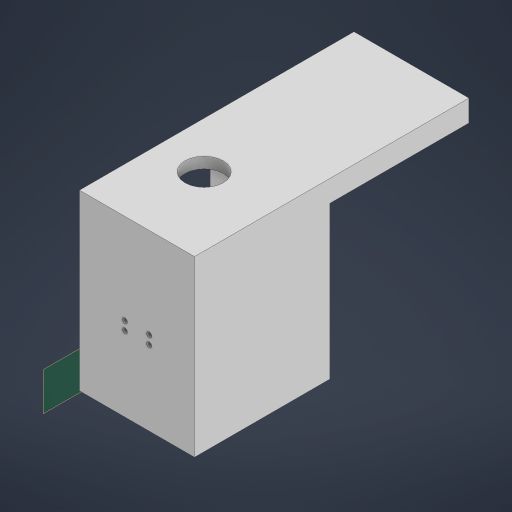
# Autodesk Inventor part: Gearbox
Saved by Autodesk Inventor 2024 (Build 280153000, 153)
## iProperties
Created: 2024-03-09
Part Number: Gearbox
Material: Generic
Document SubType Name: Modeling
Designer: LightStore
Density: 1 g/cm^3
Appearance: Default
Author: LightStore
Autodesk Inventor part; units mm, degrees
ref_plane "YZ Plane" through (0, 0, 0) normal (1, 0, 0) x (0, 1, 0)
ref_plane "XZ Plane" through (0, 0, 0) normal (0, 1, 0) x (-1, 0, 0)
ref_plane "XY Plane" through (0, 0, 0) normal (0, 0, 1) x (1, 0, 0)
sketch "Sketch1" plane through (0, 0, 0) normal (0, 0, 1) x (1, 0, 0)
  line L0 (-24.7628, 24.1619) -> (95.2372, 24.1619)
  line L1 (95.2372, 24.1619) -> (95.2372, -75.8381)
  line L2 (95.2372, -75.8381) -> (-24.7628, -75.8381)
  line L3 (-24.7628, -75.8381) -> (-24.7628, 24.1619)
  point P0 (0, 0)
  dimension "d0" = 120
  dimension "d1" = 100
  constraints: 8 end point, 2 parallel, 1 horizontal, 1 perpendicular
  measures "d0" distance of L1.end L2.end
  measures "d1" distance of L0.end L1.end
extrude "Extrusion1" add sketch "Sketch1" along normal blind 80
sketch "Sketch2" plane through (-24.7628, -75.8381, 0) normal (-1, 0, 0) x (0, 0, 1)
  line L0 (0, 0) -> (80, 0) projected
  line L1 (4.914, 93.7072) -> (77, 93.7072)
  line L2 (77, 93.7072) -> (77, 0)
  line L3 (77, 0) -> (4.914, 0)
  line L4 (4.914, 0) -> (4.914, 93.7072)
  line L5 (80, 100) -> (80, 0) projected
  line L6 (0, 100) -> (0, 0) projected
  point P0 (0, 75.8381)
  point P1 (4.914, 0)
  dimension "d6" = 3
  dimension "d108" = 4.914
  constraints: 8 end point, 2 parallel, 1 horizontal, 1 perpendicular, 1 point on line
  measures "d6" distance between parallel lines of L2 L5
  measures "d108" distance between parallel lines of L6 L4
extrude "Extrusion2" cut sketch "Sketch2" against normal blind 60
sketch "Sketch3" plane through (-24.7628, 24.1619, 0) normal (0, 1, 0) x (1, 0, 0)
  line L0 (0, 0) -> (0, -4.914) projected
  line L1 (0, 0) -> (0, -31.38)
  circle A0 centre (26.718, -35) radius 11
  line L2 (120, 0) -> (0, 0) projected
  point P0 (24.7628, 0)
  dimension "d7" = 31.38
  dimension "d9" = 22
  dimension "d109" = 35
  constraints: 2 end point, 1 centre point, 1 collinear
  measures "d7" distance of L0.start L1.end
  measures "d9" diameter of A0
  measures "d109" distance from line of L2 A0.centre
extrude "Extrusion3" cut sketch "Sketch3" against normal blind 80
sketch "Sketch8" plane through (0, 0, 0) normal (0, 0, -1) x (-1, 0, 0)
  line L0 (-95.2372, 24.1619) -> (24.7628, 24.1619) projected
  line L1 (-1.9784, 24.1619) -> (-38.1484, 24.1619)
  circle A0 centre (-1.7434, -26.1683) radius 3.5
  circle A1 centre (-10.4934, -46.1683) radius 1.575
  circle A2 centre (7.0066, -46.1683) radius 1.575
  line L2 (7.0066, -46.1683) -> (-10.4934, -46.1683)
  line L3 (-1.7434, -26.1683) -> (-1.7434, -46.1683)
  point P0 (0, 0)
  point P1 (-4.8068, -28.0128)
  dimension "d26" = 36.17
  dimension "d143" = 3.15
  dimension "d144" = 3.15
  dimension "d145" = 20
  constraints: 6 end point, 3 centre point, 2 point on line, 1 coincident, 1 horizontal, 1 midpoint
  measures "d26" distance of L1.start L1.end
  measures "d143" diameter of A1
  measures "d144" diameter of A2
  measures "d145" distance of L3.start L3.end
sketch "Sketch9" plane through (0, 0, 80) normal (0, 0, 1) x (1, 0, 0)
  line L0 (95.2372, 24.1619) -> (-24.7628, 24.1619) projected
  line L1 (41.408, 24.1619) -> (95.2372, 24.1619)
  line L2 (95.2372, 24.1619) -> (95.2372, -75.6591)
  line L3 (95.2372, -75.6591) -> (41.408, -75.6591)
  line L4 (41.408, -75.6591) -> (41.408, 24.1619)
  point P0 (0, 0)
  constraints: 8 end point, 2 parallel, 1 horizontal, 1 perpendicular, 1 point on line
extrude "Extrusion8" cut sketch "Sketch9" against normal blind 82.75
sketch "Sketch11" plane through (41.408, -75.6591, 80) normal (0, 1, 0) x (1, 0, 0)
  line L0 (0, 0) -> (-66.1708, 0) projected
  line L1 (-66.1708, 80) -> (53.8292, 80) projected
  line L2 (0, 0) -> (53.8292, 0)
  line L3 (53.8292, 0) -> (53.8292, 80)
  line L4 (53.8292, 80) -> (0, 80)
  line L5 (0, 80) -> (0, 0)
  point P0 (-41.408, 80)
  constraints: 8 end point, 2 parallel, 1 horizontal, 1 perpendicular
extrude "Extrusion9" cut sketch "Sketch11" against normal blind 82.75
sketch "Sketch16" plane through (-24.7628, -75.8381, 77) normal (0, -1, 0) x (1, 0, 0)
  line L0 (0, -72.086) -> (0, 0) projected
  line L1 (0, 0) -> (60, 0) projected
  line L2 (0, -72.086) -> (60, -72.086)
  line L3 (60, -72.086) -> (60, 0)
  line L4 (60, 0) -> (0, 0)
  line L5 (0, 0) -> (0, -72.086)
  circle A0 centre (26.718, -42) radius 11 projected
  circle A1 centre (26.718, -42) radius 5
  point P0 (24.7628, -77)
  constraints: 8 end point, 2 parallel, 1 centre point, 1 coincident, 1 horizontal, 1 perpendicular
extrude "Extrusion14" add sketch "Sketch16" against normal blind 10 contours L0 L1 L3 L2
ref_plane "Work Plane1" through (-34.7628, -75.8381, 80) normal (-1, 0, 0) x (0, 0, 1)
sketch "Sketch24" plane through (-34.7628, -75.8381, 80) normal (-1, 0, 0) x (0, 0, 1)
  line L0 (-131.9676, 100) -> (-77.9351, 100)
  line L1 (-77.9351, 100) -> (-77.9351, -1.253)
  line L2 (-77.9351, -1.253) -> (-131.9676, -1.253)
  line L3 (-131.9676, -1.253) -> (-131.9676, 100)
  point P0 (-80, 75.8381)
  constraints: 8 end point, 2 parallel, 1 horizontal, 1 perpendicular
extrude "Extrusion19" cut sketch "Sketch24" against normal blind 103.25
sketch "Sketch27" plane through (0, 0, 80) normal (0, 0, 1) x (1, 0, 0)
  line L0 (-24.7628, -75.8381) -> (41.408, -75.8381) projected
  circle A0 centre (15.3226, -32.8381) radius 1.5
  line L1 (15.3226, -32.8381) -> (1.3226, -32.8381)
  line L2 (15.3226, -35.3779) -> (15.3226, -32.8381)
  circle A1 centre (15.3226, -27.8381) radius 1.5
  circle A2 centre (1.3226, -32.8381) radius 1.5
  circle A3 centre (1.3226, -27.8381) radius 1.5
  line L3 (41.408, 24.1619) -> (-24.7628, 24.1619) projected
  point P0 (0, 0)
  dimension "d125" = 5
  dimension "d128" = 14
  dimension "d169" = 52
  constraints: 4 centre point, 4 end point, 2 horizontal, 1 vertical, 6 other
  measures "d125" distance of L1.start A1.centre
  measures "d128" distance of L1.start A2.centre
  measures "d169" distance from line of A3.centre L3
extrude "Extrusion22" cut sketch "Sketch27" against normal blind 20
extrude "Extrusion24" cut sketch "Sketch8" against normal blind 10
sketch "Sketch28" plane through (41.408, 24.1619, 2.0649) normal (0, 0, -1) x (-1, 0, 0)
  line L0 (0, -100) -> (0, 0) projected
  line L1 (66.1708, -90) -> (66.1708, -6.2928) projected
  line L2 (0, 0) -> (66.1708, 0)
  line L3 (66.1708, 0) -> (66.1708, -12.3951)
  line L4 (66.1708, -12.3951) -> (0, -12.3951)
  line L5 (0, -12.3951) -> (0, 0)
  point P0 (41.408, -24.1619)
  point P1 (0, -12.3951)
  constraints: 8 end point, 2 parallel, 1 horizontal, 1 perpendicular, 1 point on line
extrude "Extrusion25" add sketch "Sketch28" along normal blind 80
sketch "Sketch29" plane through (-24.7628, 11.7668, 2.0649) normal (0, -1, 0) x (1, 0, 0)
  line L0 (66.1708, -80) -> (0, -80) projected
  line L1 (66.1708, -80) -> (66.1708, -78.32)
  line L2 (66.1708, 0) -> (66.1708, -80) projected
  circle A0 centre (56.4908, -78.32) radius 0.75
  line L3 (56.4908, -78.32) -> (13.4908, -78.32)
  line L4 (56.4908, -61.93) -> (56.4908, -78.32)
  circle A1 centre (13.4908, -78.32) radius 0.75
  circle A2 centre (56.4908, -60.32) radius 0.75
  circle A3 centre (13.4908, -60.32) radius 0.75
  point P0 (24.7628, -2.0649)
  dimension "d150" = 1.5
  dimension "d155" = 43
  dimension "d158" = 18
  dimension "d163" = 18
  constraints: 6 end point, 4 centre point, 2 horizontal, 1 point on line, 1 vertical, 6 other
  measures "d150" diameter of A0
  measures "d155" distance of L3.start A1.centre
  measures "d158" distance of L3.start A2.centre
  measures "d163" distance of L3.end A3.centre
extrude "Extrusion26" cut sketch "Sketch29" against normal blind 10
sketch "Sketch30" plane through (-24.7628, 11.7668, 2.0649) normal (0, -1, 0) x (1, 0, 0)
  circle A0 centre (56.4908, -78.32) radius 0.75 projected
  line L0 (0, -80) -> (66.1708, -80) projected
  line L1 (43.4258, -80) -> (25.7382, -80)
  line L2 (25.7382, -80) -> (25.7382, -75)
  line L3 (25.7382, -75) -> (43.4258, -75)
  line L4 (43.4258, -75) -> (43.4258, -80)
  point P0 (24.7628, -2.0649)
  point P1 (25.7382, -80)
  point P2 (43.4258, -80)
  dimension "d165" = 5
  dimension "d168" = 13.065
  constraints: 8 end point, 2 parallel, 1 horizontal, 1 perpendicular
  measures "d165" distance of L3.end L1.start
  measures "d168" distance from line of L4 A0.centre
extrude "Extrusion27" cut sketch "Sketch30" against normal blind 6 contours L2 L3 L4 L0
body "Solid1"
